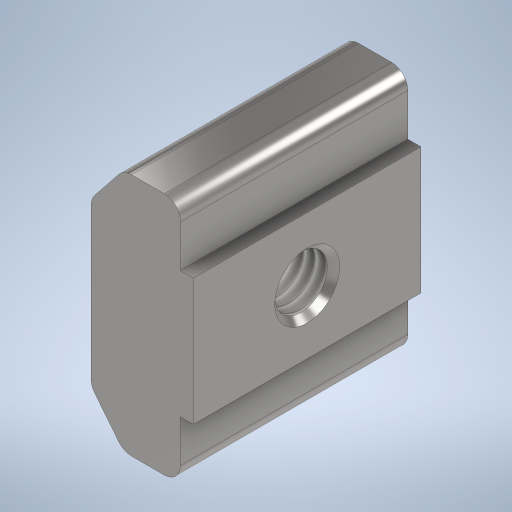
# Autodesk Inventor part: HNTT6-4
Saved by Autodesk Inventor 2024 (Build 280153000, 153)
## iProperties
Category: PARTsolutions
Company: MISUMI
Created: 2024-12-13
Part Number: HNTT6-4
Material: ステンレス鋼
Catalog Web Link: www.cadenas.de
Description: HNTT6, HNTTV6, HNTTZ6, HNTTSN6, HNTTSS6-Pre-Assembly Insertion Nuts for Aluminum Extrusions - Standard -HFS6 Series (Aluminum Extrusions 30, 50, 60, 100 Square)-
Vendor: MISUMI
Document SubType Name: Modeling
Designer: psAdmin
Manufacturer: MISUMI
Mass: 8.89184 g
Surface Area: 7.55394 cm^2
Volume: 1.11148 cm^3
Density: 8 g/cm^3
Appearance: 半つや出し
PSOL_IDENT_0: {$CADENAS_DATA/23d-libs/misumi/metric/38_al_extrusions_blackets/nuts/hntt6.prj},188 {VTYP=3D},{NB=HN
PSOL_IDENT_1: TT6-4},{LINA=HNTT6-4},{NN=HNTT6, HNTTV6, HNTTZ6, HNTTSN6, HNTTSS6},{DATE=16.05.2023 02:30:03},{GEOMD
PSOL_IDENT_2: ATE=31.10.2014 05:13:00},{VERSION=},{LINEID=30},{WBVAR=M},{WBNUMERIC=}  {NB=HNTT6-4},{LINA=HNTT6-4},
PSOL_IDENT_3: {KT=DUMMY},{PN=HNTT6-4},{TYPE=HNTT6},{MAT=1010 Carbon Steel Equivalent},{M=4},{MALG= '3' , '4' , '5'
PSOL_IDENT_4: , '6' },{M3D=4},{A=7.8},{B=15.0},{E=5.5},{T=6.3},{L=14},{TT=10},{TAPER=2.000}
NB: HNTT6-4
NN: HNTT6, HNTTV6, HNTTZ6, HNTTSN6, HNTTSS6
NT: Pre-Assembly Insertion Nuts for Aluminum Extrusions - Standard -HFS6 Series (Aluminum Extrusions 30, 50, 60, 100 Square)-
NBSYN: $PN.
LINA: HNTT6-4
CATALOG: Misumi
PN: HNTT6-4
MAT: 1010 Carbon Steel Equivalent
M: 4
SUPPLIER: MISUMI
ARTICLENO: HNTT6-4
BOMINFO: HNTT6-4
CREATOR: CADENAS GmbH
Title: HNTT6-4
Author: Cadenas PARTsolutions
Comments: Pre-Assembly Insertion Nuts for Aluminum Extrusions - Standard -HFS6 Series (Aluminum Extrusions 30, 50, 60, 100 Square)-
Autodesk Inventor part; units mm, degrees
sketch "Sketch_1" plane through (0, 0, 0) normal (0, 0, 1) x (1, 0, 0)
  arc A0 (-6.3, -4.6492) -> (-6.0809, -5.2739) centre (-5.3, -4.6492) ccw
  line L0 (-6.0809, -5.2739) -> (-4.6002, -7.1247)
  arc A1 (-4.6002, -7.1247) -> (-3.8194, -7.5) centre (-3.8194, -6.5) ccw
  line L1 (-3.8194, -7.5) -> (-1.8, -7.5)
  arc A2 (-1.8, -7.5) -> (-0.8, -6.5) centre (-1.8, -6.5) ccw
  line L2 (-0.8, -6.5) -> (-0.8, -3.9)
  line L3 (-0.8, -3.9) -> (0, -3.9)
  line L4 (0, -3.9) -> (0, 3.9)
  line L5 (0, 3.9) -> (-0.8, 3.9)
  line L6 (-0.8, 3.9) -> (-0.8, 6.5)
  arc A3 (-0.8, 6.5) -> (-1.8, 7.5) centre (-1.8, 6.5) ccw
  line L7 (-1.8, 7.5) -> (-3.8194, 7.5)
  arc A4 (-3.8194, 7.5) -> (-4.6002, 7.1247) centre (-3.8194, 6.5) ccw
  line L8 (-4.6002, 7.1247) -> (-6.0809, 5.2739)
  arc A5 (-6.0809, 5.2739) -> (-6.3, 4.6492) centre (-5.3, 4.6492) ccw
  line L9 (-6.3, 4.6492) -> (-6.3, -4.6492)
  constraints: 20 end point, 12 point on circle, 6 centre point
extrude "Extrusion1" add sketch "Sketch_1" along normal mid plane 14
sketch "Sketch_5" plane through (0, 0, 0) normal (0, 0, 1) x (1, 0, 0)
  line L0 (0, 0) -> (-6.3, 0)
  line L1 (-6.3, 0) -> (-6.3, 2)
  line L2 (-6.3, 2) -> (-5.921, 1.621)
  line L3 (-5.921, 1.621) -> (-0.379, 1.621)
  line L4 (-0.379, 1.621) -> (0, 2)
  line L5 (0, 2) -> (0, 0)
  line L6 (0, 0) -> (-6.3, 0)
  constraints: 14 end point
revolve "Revolution1" cut sketch "Sketch_5" angle 360 about axis through (0, 0, 0) along (1, 0, 0)
thread "Thread1" size "M4x0.7" class "6H" standard "ISO Metric profile" full length
ref_plane "nut_XY" through (0, 0, 0) normal (1, 0, 0) x (0, 0, -1)
ref_plane "nut_YZ" through (0, 0, 0) normal (0, 0, -1) x (0, 1, 0)
ref_plane "nut_ZX" through (0, 0, 0) normal (0, 1, 0) x (1, 0, 0)
ref_plane "to_bolt_XY" through (-6.3, 0, 0) normal (1, 0, 0) x (0, 0, -1)
ref_plane "to_bolt_YZ" through (-6.3, 0, 0) normal (0, 0, -1) x (0, 1, 0)
ref_plane "to_bolt_ZX" through (-6.3, 0, 0) normal (0, 1, 0) x (1, 0, 0)
ref_plane "to_frames_XY" through (-0.8, 0, 0) normal (1, 0, 0) x (0, 0, -1)
ref_plane "to_frames_YZ" through (-0.8, 0, 0) normal (0, 0, -1) x (0, 1, 0)
ref_plane "to_frames_ZX" through (-0.8, 0, 0) normal (0, 1, 0) x (1, 0, 0)
body "Solid1"
